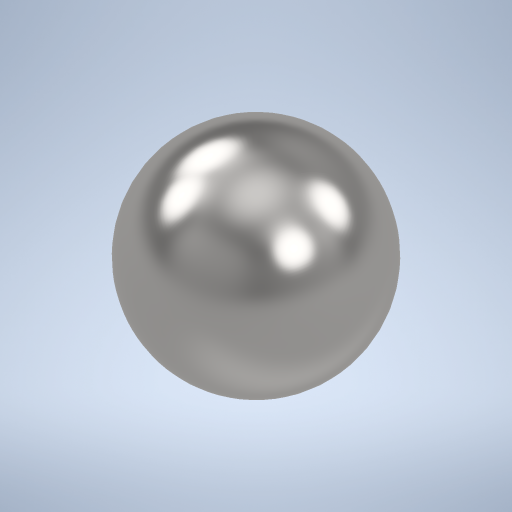
# Autodesk Inventor part: Bola
Saved by Autodesk Inventor 2024 (Build 280153000, 153)
## iProperties
Created: 2023-05-15
Part Number: Bola
Material: Aço inoxidável
Document SubType Name: Modeling
Designer: Aluno
Density: 8 g/cm^3
Appearance: Semipolido
Author: Aluno
Autodesk Inventor part; units mm, degrees
ref_plane "YZ Plane" through (0, 0, 0) normal (1, 0, 0) x (0, 1, 0)
ref_plane "XZ Plane" through (0, 0, 0) normal (0, 1, 0) x (-1, 0, 0)
ref_plane "XY Plane" through (0, 0, 0) normal (0, 0, 1) x (1, 0, 0)
sketch "Esboço1" plane through (0, 0, 0) normal (0, 0, 1) x (1, 0, 0)
  arc A0 (-9, 0) -> (9, 0) centre (0, 0) ccw
  line L0 (-9, 0) -> (9, 0)
  dimension "d0" = 18
  constraints: 2 end point, 2 point on circle, 1 centre point, 1 coincident, 1 horizontal, 1 midpoint
  measures "d0" diameter of A0
revolve "Revolução1" add sketch "Esboço1" angle 360 about axis through (-9, 0, 0) along (1, 0, 0)
